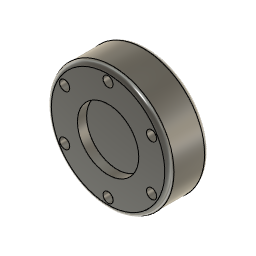
12-robo_completo (Autodesk Fusion 360 archive; units mm, degrees)
design "7-rolima"
Autodesk Fusion 360 part; units mm, degrees
sketch "Sketch1" plane through (0, 0, 0) normal (0, 1, 0) x (1, 0, 0)
  circle A0 centre (0, 0) radius 10
  circle A1 centre (0, 0) radius 20
  circle A2 centre (0, 0) radius 18.0278 construction
  circle A3 centre (-0.0049, -16.3778) radius 1.65
  line L0 (0, -22) -> (0, 22) construction
  line L1 (-25, 0) -> (28, 0) construction
  circle A4 centre (0, 0) radius 10
  circle A5 centre (0, 0) radius 10
  circle A6 centre (14.1811, -8.1931) radius 1.65
  circle A7 centre (14.186, 8.1846) radius 1.65
  circle A8 centre (0.0049, 16.3778) radius 1.65
  circle A9 centre (-14.1811, 8.1931) radius 1.65
  circle A10 centre (-14.186, -8.1846) radius 1.65
  point P0 (-0.0049, -16.3778)
  point P1 (-0.0049, 16.3778)
  dimension "d1" = 20
  dimension "d2" = 40
  dimension "d3" = 3.3
  dimension "d16" = 360
  constraint coincident A0.centre A1.centre
  constraint concentric A1 A2
  constraint tangent A2 A3
  constraint vertical L0
  constraint horizontal L1
  constraint symmetric A0 L1 A4
  constraint symmetric L1 A4 A5
  constraint coincident P0 A3.centre
  measures "d1" diameter of A0
  measures "d2" diameter of A1
  measures "d3" diameter of A3
extrude "Extrude1" add sketch "Sketch1" along normal blind 13 contours A0 A4 A5 | A1 | A3 | A6 | A7 | A8 | A9 | A10
extrude "Extrude3" cut sketch "Sketch1" along normal blind 3 contours A0 A4 A5
fillet "Fillet1" radius 1.5 2 edges at (-18.6465, 0, 7.2323) (-18.6465, 13, 7.2323)
extrude "Extrude4" cut sketch "Sketch1" along normal blind 8 contours A3 | A6 | A7 | A8 | A9 | A10
sketch "Sketch2" plane through (0, 13, 0) normal (0, 1, 0) x (-1, 0, 0)
  circle A0 centre (0, 0) radius 18.5
  circle A1 centre (0, 0) radius 18
  dimension "d17" = 36
  constraint concentric A0 A1
  measures "d17" diameter of A1
extrude "Extrude5" cut sketch "Sketch2" against normal blind 3 contours A1

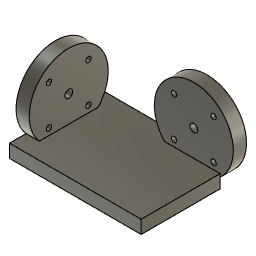
design "4-conexao_braco_punho"
Autodesk Fusion 360 part; units mm, degrees
sketch "Sketch1" plane through (0, 0, 0) normal (0, 0, 1) x (1, 0, 0)
  line L0 (-25, 50) -> (75, 50)
  line L1 (75, 50) -> (75, -20)
  line L2 (75, -20) -> (-25, -20)
  line L3 (-25, -20) -> (-25, 50)
  dimension "d1" = 100
  dimension "d2" = 70
  constraint horizontal L0
  constraint vertical L1
  constraint horizontal L2
  constraint vertical L3
  measures "d1" distance of L0.start L0.end
  measures "d2" distance of L0.start L2.end
extrude "Extrude1" add sketch "Sketch1" along normal blind 10
sketch "Sketch2" plane through (0, 0, 0) normal (1, 0, 0) x (0, 1, 0)
  line L0 (-20, 50) -> (-20, -25) construction
  line L1 (50, 50) -> (50, -25) construction
  line L2 (-25, 0) -> (55, 0) construction
  line L3 (15, 50) -> (15, -25) construction
  line L4 (-25, 30) -> (55, 30) construction
  circle A0 centre (15, 30) radius 3
  circle A1 centre (15, 30) radius 30
  circle A2 centre (0, 15) radius 2
  circle A3 centre (15, 30) radius 3
  circle A4 centre (0, 45) radius 2
  circle A5 centre (30, 45) radius 2
  circle A6 centre (15, 30) radius 3
  circle A7 centre (30, 15) radius 2
  circle A8 centre (15, 30) radius 3
  line L5 (59.9207, 15) -> (-20, 15) construction
  line L6 (30, 60) -> (30, -2) construction
  line L7 (0, 60) -> (0, -2) construction
  point P0 (0, 45)
  dimension "d5" = 35
  dimension "d6" = 30
  dimension "d7" = 6
  dimension "d8" = 60
  dimension "d9" = 4
  dimension "d10" = 4
  dimension "d18" = 15
  dimension "d19" = 15
  constraint vertical L0
  constraint vertical L1
  constraint perpendicular L1 L2
  constraint perpendicular L2 L3
  constraint perpendicular L1 L4
  constraint concentric A0 A1
  constraint symmetric L4 A0 A3
  constraint symmetric L4 A2.centre P0
  constraint coincident P0 A4.centre
  constraint symmetric L3 A3 A6
  constraint symmetric L3 A4 A5
  constraint symmetric L3 A2 A7
  constraint symmetric L3 A3 A8
  constraint coincident L0 L5.end
  constraint perpendicular L0 L5
  constraint perpendicular L2 L6
  constraint perpendicular L2 L7
  measures "d5" distance of L0 L3
  measures "d6" distance of L2 L4
  measures "d7" diameter of A0
  measures "d8" diameter of A1
  measures "d9" diameter of A2
  measures "d10" diameter of A4
  measures "d18" distance of L4 L5
  measures "d19" distance of L3 L7
extrude "Extrude2" add sketch "Sketch2" along normal blind 10 from surface at -25 contours A1 | A2 | A4 | A5 | A7
sketch "Sketch3" plane through (0, 0, 0) normal (0, 1, 0) x (1, 0, 0)
  line L0 (-30, 0) -> (80, 0) construction
  line L1 (25, -65) -> (25, 5) construction
  line L2 (-30, -30) -> (80, -30) construction
  line L3 (-25, -65) -> (-25, 5) construction
  line L4 (-35, -15) -> (111.1834, -15) construction
  line L5 (55, -65) -> (55, 5) construction
  line L6 (70, -70) -> (70, 15) construction
  circle A0 centre (55, -30) radius 30
  circle A1 centre (40, -45) radius 2
  circle A2 centre (55, -30) radius 3
  circle A3 centre (70, -45) radius 2
  circle A4 centre (40, -15) radius 2
  circle A5 centre (70, -15) radius 2
  point P0 (70, -15)
  dimension "d14" = 50
  dimension "d15" = 30
  dimension "d20" = 15
  dimension "d21" = 15
  dimension "d53" = 4
  constraint horizontal L0
  constraint perpendicular L0 L1
  constraint horizontal L2
  constraint perpendicular L0 L3
  constraint horizontal L4
  constraint perpendicular L0 L5
  constraint vertical L6
  constraint coincident P0 A5.centre
  measures "d14" distance of L1 L3
  measures "d15" distance of L0 L2
  measures "d20" distance of L2 L4
  measures "d21" distance of L5 L6
  measures "d53" diameter of A5
extrude "Extrude3" add sketch "Sketch3" against normal blind 10 from surface at 50 contours A0 | A1 | A3 | A4 | A5
ref_plane "WorkPlane1" through (0, -30, 0) normal (0, 1, 0) x (0, 0, 1)
sketch "Sketch4" plane through (0, -30, 0) normal (0, 1, 0) x (1, 0, 0)
  line L0 (85, 0) -> (-35, 0) construction
  line L1 (-35, -7.64) -> (92.4851, -7.64) construction
  line L2 (55, -30) -> (55, 12) construction
  line L3 (25, -75) -> (25, 12.7577) construction
  line L4 (75.0008, -7.64) -> (75.0008, 2)
  circle A0 centre (55, -30) radius 30
  line L5 (88, 0) -> (48, 0)
  constraint horizontal L0
  constraint horizontal L1
  constraint perpendicular L1 L2
  constraint vertical L3
extrude "Extrude6" cut sketch "Sketch4" against normal blind 10 from surface at 80 contours L4 A0 L5
extrude "Extrude8" cut sketch "Sketch2" against normal blind 8 from surface at -15 contours A2 | A4 | A5 | A7
extrude "Extrude9" cut sketch "Sketch3" along normal blind 8 from surface at 40 contours A1 | A3 | A4 | A5

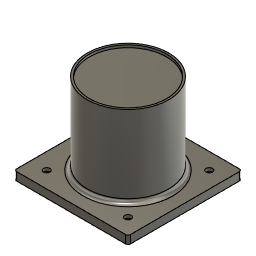
design "1-base"
Autodesk Fusion 360 part; units mm, degrees
sketch "Sketch1" plane through (0, 0, 0) normal (0, 1, 0) x (1, 0, 0)
  line L0 (70, -70) -> (-70, -70)
  line L1 (-70, -70) -> (-70, 70)
  line L2 (-70, 70) -> (70, 70)
  line L3 (70, 70) -> (70, -70)
  line L4 (70, -70) -> (-70, 70) construction
  line L5 (-70, -70) -> (70, 70) construction
  dimension "d1" = 140
  dimension "d2" = 140
  constraint horizontal L0
  constraint perpendicular L0 L1
  constraint parallel L0 L2
  constraint parallel L1 L3
  constraint coincident L4 origin
  constraint coincident L5 origin
  measures "d1" distance of L1.end L2.end
  measures "d2" distance of L0.end L1.end
extrude "Extrude1" add sketch "Sketch1" along normal blind 10
sketch "Sketch2" plane through (0, 10, 0) normal (0, 1, 0) x (-1, 0, 0)
  line L0 (-70, -70) -> (70, -70)
  line L1 (70, -70) -> (70, 70)
  line L2 (70, 70) -> (-70, 70)
  line L3 (-70, 70) -> (-70, -70)
  circle A0 centre (0, 0) radius 50
  dimension "d5" = 100
  constraint coincident A0.centre origin
  measures "d5" diameter of A0
extrude "Extrude2" add sketch "Sketch2" along normal blind 100 contours A0
sketch "Sketch3" plane through (0, 0, 0) normal (0, 0, 1) x (1, 0, 0)
  line L0 (-40, 80) -> (40, 80)
  line L1 (40, 80) -> (40, 40)
  line L2 (40, 40) -> (-40, 40)
  line L3 (-40, 40) -> (-40, 80)
  dimension "d8" = 80
  dimension "d9" = 40
  dimension "d10" = 40
  dimension "d11" = 40
  constraint horizontal L0
  constraint vertical L1
  constraint horizontal L2
  constraint vertical L3
  measures "d8" distance of L0.start L0.end
  measures "d9" distance of L0.start L2.end
  measures "d10" horizontal distance of origin L2.end
  measures "d11" distance of origin L2
sketch "Sketch4" plane through (0, 110, 0) normal (0, 1, 0) x (-1, 0, 0)
  circle A0 centre (0, 0) radius 50
  circle A1 centre (0, 0) radius 47.5
  dimension "d14" = 95
  constraint coincident A0.centre A1.centre
  measures "d14" diameter of A1
extrude "Extrude4" cut sketch "Sketch4" against normal blind 3 contours A1
sketch "Sketch5" plane through (0, 10, 0) normal (0, 1, 0) x (-1, 0, 0)
  circle A0 centre (0, 0) radius 50
  line L0 (-70, -70) -> (70, -70)
  line L1 (70, -70) -> (70, 70)
  line L2 (70, 70) -> (-70, 70)
  line L3 (-70, 70) -> (-70, -70)
  point P0 (50, -50)
  point P1 (-50, -50)
  point P2 (-50, 50)
  point P3 (50, 50)
  dimension "d17" = 20
  dimension "d18" = 20
  dimension "d19" = 20
  dimension "d20" = 20
  dimension "d21" = 20
  dimension "d22" = 20
  dimension "d23" = 20
  dimension "d24" = 20
  measures "d17" horizontal distance of L0.end P0
  measures "d18" vertical distance of L0.end P0
  measures "d19" horizontal distance of L0.start P1
  measures "d20" vertical distance of L0.start P1
  measures "d21" horizontal distance of L2.end P2
  measures "d22" vertical distance of L2.end P2
  measures "d23" horizontal distance of L1.end P3
  measures "d24" vertical distance of L1.end P3
hole "Hole1" at (50, 10, -50) at (-50, 10, -50) at (-50, 10, 50) at (50, 10, 50) direction (0, -1, 0) diameter 4.5 depth 40 tip angle 118 counterbore diameter 8 counterbore depth 4
fillet "Fillet1" radius 3 4 edges at (70, 5, 70) (-70, 5, 70) (70, 5, -70) (-70, 5, -70)
fillet "Fillet4" radius 5 1 edges at (46.6164, 10, 18.0808)
